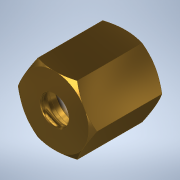
# Autodesk Inventor part: MINI-swivel-nut
Saved by Autodesk Inventor 2021 (Build 250183000, 183)
## iProperties
Company: Prusa Development a.s.
Created: 2019-10-03
Material: Všeobecné
Document SubType Name: Modeling
Density: 1 g/cm^3
Appearance: Mosaz – leštěná
Project: ORIGINAL PRUSA MINI
Authority: Ing. Robert Turinský
Author: Ing. Robert Turinský
Revision Number: R4
Autodesk Inventor part; units mm, degrees
ref_plane "YZ Plane" through (0, 0, 0) normal (1, 0, 0) x (0, 1, 0)
ref_plane "XZ Plane" through (0, 0, 0) normal (0, 1, 0) x (-1, 0, 0)
ref_plane "XY Plane" through (0, 0, 0) normal (0, 0, 1) x (1, 0, 0)
sketch "Náčrt1" plane through (0, 0, 0) normal (0, 1, 0) x (-1, 0, 0)
  line L0 (1.5, 0) -> (-9, 0) projected
  line L1 (0, -2.08) -> (0, 12.48) projected
  line L2 (-2.05, 10.3) -> (-2.05, 10)
  line L3 (-2.05, 10.3) -> (-2.15, 10.4)
  line L4 (-2.15, 10.4) -> (-5, 10.4)
  line L5 (-5, 10.4) -> (-5, 0)
  line L6 (-5, 0) -> (-3.46, 0)
  arc A0 (-3.5, 8.55) -> (-2.05, 10) centre (-3.5, 10) ccw
  line L7 (-3.46, 0) -> (-3.46, 7.0477)
  line L8 (-3.46, 7.0477) -> (-3.75, 7.55)
  line L9 (-3.75, 7.55) -> (-3.75, 8.55)
  line L10 (-3.5, 8.55) -> (-3.75, 8.55)
  line L11 (-5, 10.4) -> (-7.5, 10.4)
  line L12 (-7.5, 10.4) -> (-7.5, 8.9566)
  line L13 (-7.5, 8.9566) -> (-5, 10.4)
  line L14 (-5, 0) -> (-7.5, 0)
  line L15 (-7.5, 0) -> (-7.5, 1.4434)
  line L16 (-7.5, 1.4434) -> (-5, 0)
  line L17 (-3.46, 7.0477) -> (-3.46, 8.5506)
  point P0 (0, 0)
  dimension "d0" = 4.1
  dimension "d1" = 1.45
  dimension "d3" = 6.92
  dimension "d5" = 10
  dimension "d6" = 7.5
  dimension "d7" = 30
  dimension "d8" = 1
  dimension "d9" = 0.1
  dimension "d10" = 45
  dimension "d11" = 0.4
  dimension "d12" = 10.4
  dimension "d13" = 30
  dimension "d14" = 15
  constraints: 32 end point, 5 point on line, 4 perpendicular, 3 point on circle, 2 tangent, 2 vertical, 1 centre point, 1 collinear, 1 equal length, 1 horizontal, 1 parallel
  measures "d0" diameter of L2 L1
  measures "d1" radius of A0
  measures "d3" diameter of L7 L1
  measures "d5" diameter of L5 L1
  measures "d6" diameter of L9 L1
  measures "d7" angle of L1 L8
  measures "d8" distance of L8.end L9.end
  measures "d9" horizontal distance of L2.start L3.end
  measures "d10" angle of L4 L3
  measures "d11" distance from line of L2.end L4
  measures "d12" distance between parallel lines of L0 L4
  measures "d13" angle of L11 L13
  measures "d14" diameter of L12 L1
revolve "Rotace1" add sketch "Náčrt1" angle 360 about axis through (0, 0, -10) along (0, 0, 1) contours L0 L5 L4 L3 L2 A0 L10 L9 L8 L7 | L8 L9 L10 A0 L17
thread "Závit1" size "M8x1" class "6H" standard "ANSI Metric M Profile" length 7.55
sketch "Náčrt2" plane through (0, 0, 0) normal (0, 0, 1) x (1, 0, 0)
  circle A0 centre (0, 0) radius 5 projected
  circle A1 centre (0, 0) radius 5 projected
  line L0 (-5.7735, 0) -> (-2.8868, 5)
  line L1 (-2.8868, 5) -> (2.8868, 5)
  line L2 (2.8868, 5) -> (5.7735, 0)
  line L3 (5.7735, 0) -> (2.8868, -5)
  line L4 (2.8868, -5) -> (-2.8868, -5)
  line L5 (-2.8868, -5) -> (-5.7735, 0)
  dimension "d16" = 10
  constraints: 12 end point, 1 coincident, 1 horizontal, 13 other
  measures "d16" distance between parallel lines of L4 L1
extrude "Vysunutí1" add sketch "Náčrt2" along normal blind 10.4 contours A0 L2 L3 | A0 L1 L2 | L3 L4 A0 | A0 L0 L1 | L4 L5 A0 | A0 L5 L0
revolve "Rotace2" cut sketch "Náčrt1" angle 360 about axis through (0, 0, -10) along (0, 0, 1) contours L0 L15 L16 | L13 L12 L11
revolve "Rotace3" cut sketch "Náčrt1" angle 360 about axis through (0, 0, -10) along (0, 0, 1) contours L8 L9 L10 A0 L17
chamfer "Zkosení1" distance 0.75 angle 45 1 edges at (-3.46, 0, 0)
equation "\"d17\" = d12"
